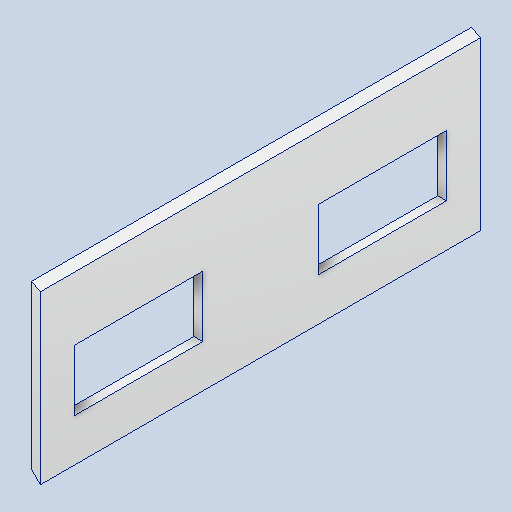
# Autodesk Inventor part: plug_nowy
Saved by Autodesk Inventor 2023 (Build 270158000, 158)
## iProperties
Created: 2023-07-07
Part Number: plug_nowy
Material: Aluminium 6061
Document SubType Name: Modeling
Designer: Kamil
Density: 2.7 g/cm^3
Appearance: Aluminium — płaski
Author: Kamil
Autodesk Inventor part; units mm, degrees
ref_plane "YZ Plane" through (0, 0, 0) normal (1, 0, 0) x (0, 1, 0)
ref_plane "XZ Plane" through (0, 0, 0) normal (0, 1, 0) x (-1, 0, 0)
ref_plane "XY Plane" through (0, 0, 0) normal (0, 0, 1) x (1, 0, 0)
sketch "Szkic1" plane through (0, 0, 0) normal (1, 0, 0) x (0, 1, 0)
  line L0 (9.1767, 36.8868) -> (23.0303, 36.8868)
  line L1 (23.0303, 36.8868) -> (23.0303, 8.0794)
  line L2 (22.5303, 5.7086) -> (9.1767, 5.7086)
  line L3 (9.1767, 5.7086) -> (9.1767, 36.8868)
  line L4 (0, 100) -> (39.1311, 100)
  line L5 (39.1311, 0) -> (0, 0)
  line L6 (23.0303, 63.1132) -> (9.1767, 63.1132)
  line L7 (9.1767, 63.1132) -> (9.1767, 94.2914)
  line L8 (9.1767, 94.2914) -> (23.0303, 94.2914)
  line L9 (23.0303, 94.2914) -> (23.0303, 63.1132)
  line L10 (39.1311, 100) -> (40.1311, 100)
  line L11 (40.1311, 0) -> (39.1311, 0)
  line L12 (40.1311, 100) -> (40.1311, 0)
  line L13 (-0.559, 100) -> (-0.1118, 100)
  line L14 (-0.559, 100) -> (-0.559, 0)
  line L15 (-0.1118, 0) -> (-0.559, 0)
  line L16 (-0.1118, 100) -> (0.1125, 100)
  line L17 (23.0303, 8.0794) -> (23.0303, 5.7086)
  line L18 (23.0303, 5.7086) -> (22.5303, 5.7086)
  line L19 (40.1311, 100) -> (-0.559, 100)
  line L20 (-0.559, 100) -> (-0.559, 0)
  line L21 (-0.559, 0) -> (40.1311, 0)
  line L22 (40.1311, 0) -> (40.1311, 100)
  point P0 (11.7487, 100)
  constraints: 46 end point, 2 parallel, 1 collinear, 1 horizontal, 1 perpendicular, 1 point on line, 1 vertical
extrude "Wyciągnięcie proste1" add sketch "Szkic1" along normal blind 2
chamfer "Faza1" distance 2 angle 45 2 edges at (0, -0.559, 50) (2, 40.1311, 50)
sketch "Szkic2" plane through (0, 1.441, 100) normal (0, 0, 1) x (1, 0, 0)
  line L0 (0, 37.0479) -> (-58.736, 68.461) projected
  line L1 (0, 37.0479) -> (5, 34.3738)
  line L2 (5, 34.3738) -> (2.5, 39)
  line L3 (2.5, 39) -> (-2, 40)
  line L4 (-2, 40) -> (-2.3739, 38.3175)
  point P0 (0, -1.441)
  constraints: 8 end point, 1 collinear, 1 perpendicular, 1 point on line
extrude "Wyciągnięcie proste2" cut sketch "Szkic2" against normal through all
sketch "Szkic3" plane through (2, 0, 0) normal (1, 0, 0) x (0, 0, -1)
  line L0 (-94.2914, 9.1767) -> (-94.2914, 23.0303) projected
  line L1 (-94.2914, 23.0303) -> (-63.1132, 23.0303) projected
  line L2 (-63.1132, 9.1767) -> (-94.2914, 9.1767) projected
  line L3 (-5.7086, 9.1767) -> (-36.8868, 9.1767) projected
  line L4 (-36.8868, 23.0303) -> (-5.7086, 23.0303) projected
  line L5 (-5.7086, 23.0303) -> (-5.7086, 9.1767) projected
  line L6 (-63.1132, 9.1767) -> (-94.2914, 9.1767) projected
  line L7 (-94.2914, 23.0303) -> (-92.2914, 23.0303)
  line L8 (-92.2914, 23.0303) -> (-92.2914, 9.1767)
  line L9 (-92.2914, 9.1767) -> (-94.2914, 9.1767)
  line L10 (-94.2914, 9.1767) -> (-94.2914, 23.0303)
  line L11 (-5.7086, 9.1767) -> (-36.8868, 9.1767) projected
  line L12 (-36.8868, 23.0303) -> (-5.7086, 23.0303) projected
  line L13 (-5.7086, 9.1767) -> (-7.7086, 9.1767)
  line L14 (-7.7086, 9.1767) -> (-7.7086, 23.0303)
  line L15 (-7.7086, 23.0303) -> (-5.7086, 23.0303)
  line L16 (-5.7086, 23.0303) -> (-5.7086, 9.1767)
  point P0 (0, 0)
  dimension "d7" = 2
  dimension "d8" = 2
  constraints: 16 end point, 4 parallel, 2 horizontal, 2 perpendicular, 2 point on line
  measures "d7" distance of L8.end L9.end
  measures "d8" distance of L14.end L15.end
extrude "Wyciągnięcie proste3" add sketch "Szkic3" against normal blind 2
